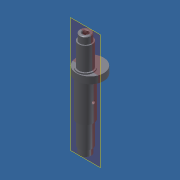
# Autodesk Inventor part: EIXO EXCÊNTRICO(53)
Saved by Autodesk Inventor 2012 SP2 (Build 160219200, 219)
## iProperties
Created: 2012-07-24
Part Number: EIXO EXCÊNTRICO(53)
Material: Carbon Steel
Document SubType Name: Modeling
Designer: bruno.silveira
Mass: 328.972 g
Surface Area: 78.7157 cm^2
Volume: 41.8008 cm^3
Density: 7.87 g/cm^3
Author: bruno.silveira
Autodesk Inventor part; units mm, degrees
ref_plane "YZ Plane" through (0, 0, 0) normal (1, 0, 0) x (0, 1, 0)
ref_plane "XZ Plane" through (0, 0, 0) normal (0, 1, 0) x (-1, 0, 0)
ref_plane "XY Plane" through (0, 0, 0) normal (0, 0, 1) x (1, 0, 0)
sketch "Sketch1" plane through (0, 0, 0) normal (0, 0, 1) x (1, 0, 0)
  circle A0 centre (0, 0) radius 12
  dimension "d0" = 24
  constraints: 1 centre point, 1 coincident
  measures "d0" diameter of A0
extrude "Extrusion1" add sketch "Sketch1" along normal blind 92.4
sketch "Sketch2" plane through (0, 0, 92.4) normal (0, 0, 1) x (1, 0, 0)
  circle A0 centre (0, 0) radius 12 projected
  circle A1 centre (0, 0) radius 5
  dimension "d3" = 10
  constraints: 1 centre point, 1 coincident
  measures "d3" diameter of A1
extrude "Extrusion2" cut sketch "Sketch2" against normal blind 6.2
sketch "Sketch3" plane through (0, 0, 86.2) normal (0, 0, 1) x (1, 0, 0)
  circle A0 centre (0, 0) radius 12 projected
  circle A1 centre (0, 0) radius 6
  dimension "d6" = 12
  constraints: 1 centre point, 1 coincident
  measures "d6" diameter of A1
extrude "Extrusion3" cut sketch "Sketch3" against normal blind 20.2
sketch "Sketch4" plane through (0, 0, 66) normal (0, 0, 1) x (1, 0, 0)
  circle A0 centre (0, 0) radius 12 projected
  circle A1 centre (0, 0) radius 7.25
  dimension "d9" = 14.5
  constraints: 1 centre point, 1 coincident
  measures "d9" diameter of A1
extrude "Extrusion4" cut sketch "Sketch4" against normal blind 1
sketch "Sketch5" plane through (0, 0, 0) normal (0, 0, -1) x (-1, 0, 0)
  circle A0 centre (0, 0) radius 12 projected
  circle A1 centre (0, 0) radius 6
  dimension "d12" = 0
  dimension "d13" = 12
  constraints: 1 centre point
  measures "d12" distance of A0.centre A1.centre
  measures "d13" diameter of A1
extrude "Extrusion5" cut sketch "Sketch5" against normal blind 26.4
sketch "Sketch6" plane through (0, 0, 0) normal (0, 0, -1) x (-1, 0, 0)
  circle A0 centre (0, 0) radius 6 projected
  circle A1 centre (0, 0) radius 5
  dimension "d16" = 10
  constraints: 1 centre point, 1 coincident
  measures "d16" diameter of A1
extrude "Extrusion6" cut sketch "Sketch6" against normal blind 6.2
sketch "Sketch7" plane through (0, 0, 26.4) normal (0, 0, -1) x (-1, 0, 0)
  circle A0 centre (0, 0) radius 6 projected
  circle A1 centre (0, 0) radius 12 projected
  circle A2 centre (0, 0) radius 7.25
  dimension "d19" = 14.5
  constraints: 1 centre point, 1 coincident
  measures "d19" diameter of A2
extrude "Extrusion7" cut sketch "Sketch7" against normal blind 32.6 contours A1
sketch "Sketch8" plane through (0, 0, 0) normal (0, 0, -1) x (-1, 0, 0)
  circle A0 centre (0, 0) radius 5 projected
hole "Hole1" at (0, 0, 0) direction (0, 0, 1) diameter 4.917 depth 18 tip angle 118 thread size "M6x1" class "6H" standard "ANSI Metric M Profile"
chamfer "Chamfer1" distance 0.5 angle 45 1 edges at (0, -2.4585, 0)
sketch "Sketch9" plane through (0, 0, 92.4) normal (0, 0, 1) x (1, 0, 0)
  circle A0 centre (0, 0) radius 5 projected
hole "Hole2" at (0, 0, 92.4) direction (0, 0, -1) diameter 4.917 depth 18 tip angle 118 thread size "M6x1" class "6H" standard "ANSI Metric M Profile"
chamfer "Chamfer2" distance 0.5 angle 45 1 edges at (0, 2.4585, 92.4)
chamfer "Chamfer3" distance 0.5 angle 45 2 edges at (-5, 0, 92.4) (5, 0, 0)
sketch "Sketch10" plane through (0, 0, 65) normal (0, 0, 1) x (1, 0, 0)
  circle A0 centre (0, 0) radius 7.25 projected
  circle A1 centre (0, 4) radius 12
  dimension "d46" = 24
  dimension "d47" = 4
  constraints: 1 centre point
  measures "d46" diameter of A1
  measures "d47" distance of A0.centre A1.centre
extrude "Extrusion8" add sketch "Sketch10" against normal blind 6
sketch "Sketch11" plane through (0, 0, 65) normal (0, 0, 1) x (1, 0, 0)
  arc A0 (-11.8322, 2) -> (11.8322, 2) centre (0, 0) ccw projected
  arc A1 (11.8322, 2) -> (-11.8322, 2) centre (0, 4) ccw projected
  circle A2 centre (0, 4) radius 12
  constraints: 1 centre point, 1 coincident
extrude "Extrusion9" cut sketch "Sketch11" against normal blind 6 contours A2 A0
sketch "Sketch13" plane through (0, 0, 0) normal (1, 0, 0) x (0, 1, 0)
  circle A0 centre (0, 42.45) radius 1.5
  line L0 (-8, 59) -> (16, 59) projected
  line L1 (-7.25, 59) -> (7.25, 59) projected
  line L2 (-7.25, 26.4) -> (7.25, 26.4) projected
  point P0 (0, 0)
  dimension "d56" = 3
  dimension "d57" = 16.55
  constraints: 1 centre point
  measures "d56" diameter of A0
  measures "d57" distance from line of L0 A0.centre
extrude "Extrusion11" cut sketch "Sketch13" along normal mid plane 20
body "Solid1"
